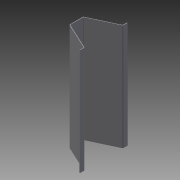
# Autodesk Inventor part: Bread Pan
Saved by Autodesk Inventor 2015 (Build 190159000, 159)
## iProperties
Created: 2016-02-06
Part Number: Bread Pan
Material: Generic
Document SubType Name: Sheet Metal
Designer: sethbattis
Density: 1 g/cm^3
Sheet Metal Rule: Default
Appearance: Default
Author: sethbattis
Autodesk Inventor part; units mm, degrees
ref_plane "YZ Plane" through (0, 0, 0) normal (1, 0, 0) x (0, 1, 0)
ref_plane "XZ Plane" through (0, 0, 0) normal (0, 1, 0) x (-1, 0, 0)
ref_plane "XY Plane" through (0, 0, 0) normal (0, 0, 1) x (1, 0, 0)
sketch "Sketch1" plane through (0, 0, 0) normal (1, 0, 0) x (0, 1, 0)
  line L0 (292.1, 38.1) -> (-292.1, 38.1)
  line L1 (-292.1, 38.1) -> (-292.1, -38.1)
  line L2 (-292.1, -38.1) -> (292.1, -38.1)
  line L3 (292.1, -38.1) -> (292.1, 38.1)
  line L4 (-408.94, 0) -> (408.94, 0)
  line L5 (0, -53.34) -> (0, 53.34)
  point P0 (0, 0)
  dimension "d0" = 76.2
  dimension "d1" = 584.2
  measures "d0" distance of L2.end L0.start
  measures "d1" distance of L1.end L2.end
extrude "Plate1" add sketch "Sketch1" along normal blind 3.048
sketch "Sketch2" plane through (1.2881, 292.1, -35.3376) normal (-0.4226183, 0, -0.9063078) x (0, -1, 0)
  line L0 (584.2, 0) -> (0, 0)
  line L1 (0, 0) -> (0, -165.1)
  line L2 (0, -165.1) -> (584.2, -165.1)
  line L3 (584.2, -165.1) -> (584.2, 0)
  constraints: 6 end point, 1 horizontal, 1 perpendicular, 1 vertical
edge flange "Flange1" height 165.1 angle 65 thickness 3.048 bend radius 3.048 thickness toward (-0.4226183, 0, -0.9063078) relief tear relief width 3.048 relief depth 1.524 corner gap 3.048 corner form 0 edges at (3.048, 0, -38.1) (3.048, 0, 38.1) wall of the first edge with corners at (1.2881, -292.1, -35.3376) (1.2881, 292.1, -35.3376) (150.9196, 292.1, -105.1118) (150.9196, -292.1, -105.1118)
bend "Bend1"
corner "Corner1"
sketch "Sketch3" plane through (147.8716, 292.1, 105.1118) normal (1, 0, 0) x (0, 1, 0)
  line L0 (-584.2, 0) -> (0, 0)
  line L1 (0, 0) -> (0, 25.4)
  line L2 (0, 25.4) -> (-584.2, 25.4)
  line L3 (-584.2, 25.4) -> (-584.2, 0)
  constraints: 6 end point, 1 horizontal, 1 perpendicular, 1 vertical
edge flange "Flange2" height 25.4 angle 65 thickness 3.048 bend radius 3.048 thickness toward (1, 0, 0) relief tear relief width 3.048 relief depth 1.524 corner gap 3.048 corner form 0 edges at (149.6314, 0, 107.8743) (149.6314, 0, -107.8743) wall of the first edge with corners at (147.8716, -292.1, 105.1118) (147.8716, 292.1, 105.1118) (147.8716, 292.1, 130.5118) (147.8716, -292.1, 130.5118)
bend "Bend2"
corner "Corner2"
equation "\"d3\" = BendReliefWidth"
equation "\"d4\" = BendReliefDepth"
equation "\"d5\" = MinimumRemnant"
equation "\"d6\" = BendRadius"
equation "\"d9\" = BendRadius"
equation "\"d10\" = CornerReliefSize"
equation "\"d11\" = GapSize"
equation "\"d12\" = JacobiRadiusSize"
equation "\"d13\" = BendReliefWidth"
equation "\"d14\" = BendReliefDepth"
equation "\"d15\" = MinimumRemnant"
equation "\"d16\" = BendRadius"
equation "\"d19\" = BendRadius"
equation "\"d20\" = CornerReliefSize"
equation "\"d21\" = GapSize"
equation "\"d22\" = JacobiRadiusSize"
equation "\"BendRadius\" = Thickness"
equation "\"BendReliefWidth\" = Thickness"
equation "\"BendReliefDepth\" = 0.5 * Thickness"
equation "\"CornerReliefSize\" = 4 * Thickness"
equation "\"MinimumRemnant\" = 2 * Thickness"
equation "\"TransitionRadius\" = BendRadius"
equation "\"JacobiRadiusSize\" = BendRadius"
equation "\"GapSize\" = Thickness"
equation "\"d2\" = BendRadius"
equation "\"Thickness\" = 3.048"
body "Solid1"
